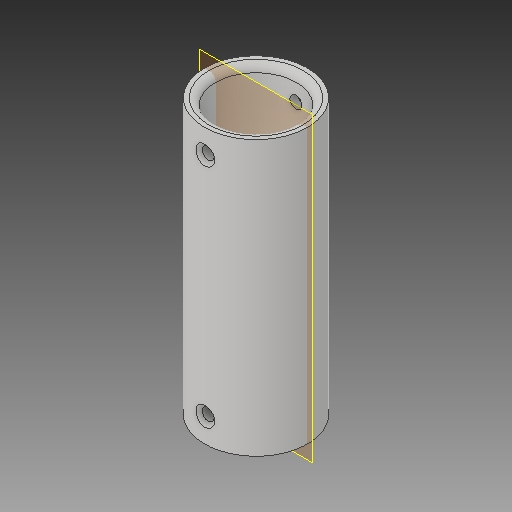
# Autodesk Inventor part: wooden_rod_joint
Saved by Autodesk Inventor 2019 (Build 230136000, 136)
## iProperties
Created: 2020-01-23
Part Number: wooden_rod_joint
Material: Generic
Document SubType Name: Modeling
Designer: Next
Density: 1 g/cm^3
Appearance: Default
Author: Next
Autodesk Inventor part; units mm, degrees
ref_plane "YZ Plane" through (0, 0, 0) normal (1, 0, 0) x (0, 1, 0)
ref_plane "XZ Plane" through (0, 0, 0) normal (0, 1, 0) x (-1, 0, 0)
ref_plane "XY Plane" through (0, 0, 0) normal (0, 0, 1) x (1, 0, 0)
sketch "Sketch1" plane through (0, 0, 0) normal (0, 1, 0) x (-1, 0, 0)
  circle A0 centre (0, 0) radius 15
  dimension "d0" = 30
  constraints: 1 centre point, 1 coincident
  measures "d0" diameter of A0
extrude "Extrusion1" add sketch "Sketch1" along normal mid plane 80
sketch "Sketch2" plane through (0, 40, 0) normal (0, 1, 0) x (1, 0, 0)
  circle A0 centre (0, 0) radius 11.75
  dimension "d3" = 23.5
  constraints: 1 centre point, 1 coincident
  measures "d3" diameter of A0
extrude "Extrusion2" cut sketch "Sketch2" against normal blind 30
sketch "Sketch3" plane through (0, -40, 0) normal (0, -1, 0) x (1, 0, 0)
  circle A0 centre (0, 0) radius 11.75
  dimension "d6" = 23.5
  constraints: 1 centre point, 1 coincident
  measures "d6" diameter of A0
extrude "Extrusion3" cut sketch "Sketch3" against normal blind 30
ref_plane "Work Plane1" through (15, 40, 0) normal (0, 0, 1) x (-1, 0, 0)
sketch "Sketch6" plane through (15, 40, 0) normal (0, 0, 1) x (-1, 0, 0)
  circle A0 centre (15, 7) radius 1.75
  line L0 (26.75, 0) -> (3.25, 0) construction
  line L1 (3.25, 0) -> (26.75, 0) construction
  circle A1 centre (15, 73) radius 1.75
  line L2 (3.25, 80) -> (26.75, 80) construction
  line L3 (3.2498, 80) -> (26.75, 80) construction
  point P0 (15, 40)
  dimension "d9" = 3.5
  dimension "d10" = 7
  dimension "d11" = 3.5
  dimension "d12" = 7
  constraints: 4 end point, 2 centre point, 1 collinear, 1 horizontal
  measures "d9" diameter of A0
  measures "d10" distance from line of A0.centre L0
  measures "d11" diameter of A1
  measures "d12" distance from line of L2 A1.centre
extrude "Extrusion4" cut sketch "Sketch6" along normal mid plane 40
fillet "Fillet1" radius 2 2 edges at (-11.75, -40, 0) (-11.75, 40, 0)
chamfer "Chamfer1" distance 1 angle 45 2 edges at (1.75, -33.0005, -14.8976) (1.75, -33.0005, 14.8976)
chamfer "Chamfer2" distance 1 angle 45 2 edges at (1.75, 32.9995, 14.8976) (1.75, 32.9995, -14.8976)
body "Solid1"
